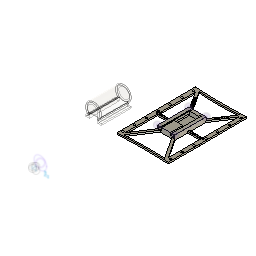
Removeable+Cap (Autodesk Fusion 360 design; units mm, degrees)
Autodesk Fusion 360 part; units mm, degrees
sketch "Sketch1" plane through (0, 0, 0) normal (0, 0, 1) x (1, 0, 0) in component "Base"
  line L0 (65.3388, 0.0001) -> (64.555, 99.997)
  arc A0 (65.3388, 0.0001) -> (0, 0) centre (32.67, -527.6145) ccw
  arc A1 (58.214, 2.2762) -> (6.5482, 1.9998) centre (35.1249, -510.6694) ccw
  arc A2 (-0.7816, 100.3921) -> (64.555, 99.997) centre (35.0771, 627.7997) ccw
  arc A3 (6.5746, 97.8855) -> (58.214, 97.7209) centre (33.5966, 474.9447) ccw
  line L1 (-0.4188, 49.9985) -> (5, 50.0245) construction
  circle A4 centre (2.2906, 50.0115) radius 1.25
  line L2 (4.7824, 95.0143) -> (-0.2636, 95.0087) construction
  circle A5 centre (2.2594, 95.0115) radius 1.25
  line L3 (2.2906, 50.0115) -> (2.274, 65.0115) construction
  line L4 (2.274, 65.0115) -> (2.2574, 80.0115) construction
  line L5 (2.2574, 80.0115) -> (2.2594, 95.0115) construction
  circle A6 centre (2.2574, 80.0115) radius 1.25
  circle A7 centre (2.274, 65.0115) radius 1.25
  circle A8 centre (62.7399, 95.0115) radius 1.25
  circle A9 centre (62.7419, 80.0115) radius 1.25
  circle A10 centre (62.7253, 65.0115) radius 1.25
  circle A11 centre (62.7087, 50.0115) radius 1.25
  circle A12 centre (62.7253, 35.0115) radius 1.25
  circle A13 centre (62.7419, 20.0115) radius 1.25
  circle A14 centre (62.7399, 5.0116) radius 1.25
  circle A15 centre (2.2594, 5.0116) radius 1.25
  circle A16 centre (2.2574, 20.0115) radius 1.25
  circle A17 centre (2.274, 35.0115) radius 1.25
  line L6 (-0.7816, 100.3921) -> (0, 0)
  line L7 (60.0224, 46.1) -> (60.0224, 5.0699)
  line L8 (5, 5) -> (5, 46.2745)
  line L9 (2.2574, 80.0115) -> (2.2576, 81.0115)
  line L10 (60.0224, 97.8257) -> (60.0224, 2.1916)
  line L11 (60.0224, 46.1) -> (60.0224, 48.6)
  line L12 (65.0224, 100) -> (65.0224, 0)
  line L13 (40.775, 30.0973) -> (72.9042, 30.0973) construction
  line L14 (60.0224, 2.1916) -> (61.5224, 2.1916) construction
  line L15 (60.0224, 2.1916) -> (61.5224, 2.1916) construction
  line L16 (58.214, 2.2762) -> (39.7178, 30.0973)
  line L17 (4.9833, 2.4465) -> (5, 2.4465) construction
  line L18 (24.6632, 30.0973) -> (6.5482, 1.9998)
  line L19 (58.214, 97.7209) -> (39.8492, 70.0973)
  line L20 (60.0224, 94.9271) -> (43.275, 69.7364)
  line L21 (24.6894, 70.0973) -> (6.5, 98)
  line L22 (5, 94.8639) -> (21.275, 69.5842)
  line L23 (64.9469, 49.9985) -> (-0.4188, 49.9985) construction
  line L24 (5, 50.0245) -> (5.0001, 49.9985)
  line L25 (5.0001, 49.9985) -> (5, 50.0245)
  line L26 (5.006, 48.7745) -> (21.275, 48.7745)
  line L27 (5, 51.2745) -> (4.994, 51.2745)
  line L28 (60.0224, 50.0087) -> (60.0224, 49.9985)
  line L29 (60.0224, 48.7587) -> (43.275, 48.9043)
  line L30 (60.0224, 94.9271) -> (60.0224, 51.2587)
  line L31 (60.0224, 48.7587) -> (60.0224, 48.6)
  line L32 (5, 49.9985) -> (5, 50.0245)
  line L33 (5, 51.2745) -> (5, 94.8639)
  line L34 (43.275, 46.4131) -> (60.0229, 46.4131)
  line L35 (60.0224, 51.2587) -> (60.0224, 48.7587)
  line L36 (21.275, 46.2745) -> (5, 46.2745)
  line L37 (4.994, 51.2745) -> (5.006, 48.7745)
  line L38 (39.8492, 70.0973) -> (24.6894, 70.0973)
  line L39 (24.6632, 30.0973) -> (39.7178, 30.0973)
  line L40 (43.275, 70.0973) -> (32.2207, 49.9985) construction
  line L41 (5, 5) -> (21.275, 30.2436)
  line L42 (60.0224, 5.0699) -> (43.275, 30.2607)
  line L43 (21.275, 70.0973) -> (32.3293, 49.9985) construction
  line L44 (21.275, 69.5842) -> (21.275, 48.7745)
  line L45 (21.275, 46.2745) -> (21.275, 30.2436)
  line L46 (43.275, 30.2607) -> (43.275, 46.4131)
  line L47 (43.275, 48.9043) -> (43.275, 69.7364)
  line L48 (43.275, 30.0973) -> (21.275, 30.0973)
  line L49 (21.275, 30.0973) -> (21.275, 70.0973)
  line L50 (21.275, 70.0973) -> (43.275, 70.0973)
  line L51 (43.275, 70.0973) -> (43.275, 30.0973)
  line L52 (43.275, 30.0973) -> (21.275, 70.0973) construction
  line L53 (21.275, 30.0973) -> (43.275, 70.0973) construction
  point P0 (32.275, 50.0973)
  point P1 (32.275, 50.0973)
  point P2 (32.275, 50.0973)
  point P3 (32.275, 50.0973)
  point P4 (32.275, 50.0973)
  dimension "d2" = 2.5
  dimension "d4" = 2.5
  dimension "d7" = 2.5
  dimension "d8" = 2.5
  dimension "d13" = 100
  dimension "d192" = 2.5
  dimension "d209" = 1
  dimension "d218" = 5
  dimension "d384" = 22
  dimension "d385" = 40
  constraint vertical L8
  constraint vertical L30
  constraint coincident A0.end L6.end
  constraint coincident L1.end L8
  constraint midpoint L1 A4.centre
  constraint midpoint L2 A5.centre
  constraint coincident A4.centre L3.start
  constraint perpendicular L2 L3
  constraint perpendicular L2 L4
  constraint coincident A5.centre L5.end
  constraint coincident L4.end L5.start
  constraint coincident L3.end L4.start
  constraint collinear L7 L30
  constraint collinear L8 L32
  constraint parallel L5 L9
  constraint coincident L10.end L14.start
  constraint horizontal L13
  constraint horizontal L14
  constraint horizontal L15
  constraint parallel L16 L42
  constraint horizontal L17
  constraint parallel L18 L41
  constraint coincident L21 A3.start
  constraint coincident P4 P3
  constraint midpoint L0 L23.start
  constraint horizontal L23
  constraint perpendicular L1 L24
  constraint perpendicular L1 L25
  constraint midpoint L10 L28.start
  constraint parallel L11 L28
  constraint collinear L30 L31
  constraint coincident L23 L28.end
  constraint coincident L23 L32.start
  constraint collinear L32 L33
  constraint coincident L23 L24.end
  constraint horizontal L34
  constraint horizontal L38
  constraint perpendicular L38 L44
  constraint parallel L38 L39
  constraint parallel L44 L46
  constraint coincident L40 P4
  constraint coincident P4 L43
  constraint coincident L23 L40.end
  constraint coincident L23 L43.end
  constraint coincident L36.start L44
  constraint coincident L29.end L46
  constraint collinear L44 L45
  constraint collinear L46 L47
  constraint horizontal L48
  constraint perpendicular L48 L49
  constraint parallel L48 L50
  constraint parallel L49 L51
  constraint coincident L52 P4
  constraint coincident L53 P4
  measures "d2" diameter of A4
  measures "d4" diameter of A5
  measures "d7" diameter of A6
  measures "d8" diameter of A7
  measures "d13" distance of L0.start L0.end
  measures "d192" diameter of A5
  measures "d209" distance of L4.end L9.end
  measures "d218" distance of L7 L12
  measures "d384" distance of L43.start L40.start
  measures "d385" distance of L48.end L43.start
extrude "Extrude1" add sketch "Sketch1" along normal blind 6 contours L38 L39 L44 L45 L46 L47 L48 L49 L50 L51 makes body 1 in component "Base"
extrude "Extrude2" add sketch "Sketch1" along normal blind 2 separate body contours L0 A0 A2 L6 L12 | L38 L39 L44 L45 L46 L47 L48 L49 L50 L51 | L10 L11 L29 L31 L34 L51 makes body 2 in component "Base"
sketch "Sketch9" plane through (0, 0, 6) normal (0, 0, 1) x (-1, 0, 0) in component "Base"
  line L0 (-23.462, -48.6115) -> (-22.275, -48.6115)
  line L1 (-32.4463, -66.0115) -> (-27.1964, -65.9812)
  line L2 (-27.1964, -65.9812) -> (-37.6964, -65.9812)
  line L3 (-23.462, -48.6115) -> (-25.9464, -48.6115)
  line L4 (-26.9547, -45.9812) -> (-22.275, -45.9812)
  line L5 (-42.275, -48.6115) -> (-38.9464, -48.6115)
  line L6 (-37.9464, -45.9812) -> (-42.275, -45.9812)
  line L7 (-42.2726, -46.1115) -> (-42.2726, -48.6115)
  line L8 (-22.275, -30.0973) -> (-42.275, -30.0973)
  line L9 (-42.275, -70.0973) -> (-22.275, -70.0973)
  line L10 (-22.462, -48.6115) -> (-22.4997, -48.6115)
  line L11 (-42.275, -48.6115) -> (-42.275, -45.9812)
  line L12 (-37.9464, -45.9812) -> (-26.9547, -45.9812)
  line L13 (-26.9464, -65.9812) -> (-37.9464, -65.9812)
  line L14 (-42.275, -70.0973) -> (-42.275, -69.0973)
  line L15 (-43.275, -70.0973) -> (-21.275, -70.0973)
  line L16 (-21.275, -70.0973) -> (-21.275, -30.0973)
  line L17 (-21.275, -30.0973) -> (-43.275, -30.0973)
  line L18 (-43.275, -30.0973) -> (-43.275, -70.0973)
  line L19 (-43.275, -70.0973) -> (-21.275, -70.0973)
  line L20 (-21.275, -70.0973) -> (-21.275, -30.0973)
  line L21 (-21.275, -30.0973) -> (-43.275, -30.0973)
  line L22 (-43.275, -30.0973) -> (-43.275, -70.0973)
  line L23 (-22.275, -45.9812) -> (-22.275, -48.6115)
  line L24 (-26.9464, -65.9812) -> (-25.9464, -65.9812)
  line L25 (-37.9464, -65.9812) -> (-38.9464, -65.9812)
  line L26 (-38.9464, -65.9812) -> (-38.9464, -45.9812)
  line L27 (-25.9464, -65.9812) -> (-25.9464, -45.9812)
  dimension "d179" = 11
  dimension "d308" = 20
  dimension "d337" = 1
  dimension "d386" = 1
  dimension "d390" = 1
  dimension "d391" = 1
  dimension "d392" = 1
  dimension "d393" = 1
  constraint horizontal L2
  constraint horizontal L3
  constraint horizontal L4
  constraint horizontal L5
  constraint horizontal L6
  constraint vertical L7
  constraint perpendicular L6 L11
  constraint coincident L9.start L14.start
  constraint coincident L6 L26.end
  constraint perpendicular L6 L26
  constraint perpendicular L24 L27
  constraint coincident L26 L5.end
  constraint coincident L27 L3.end
  constraint coincident L4 L27.end
  constraint perpendicular L4 L27
  measures "d179" distance of L13.start L13.end
  measures "d308" distance of L2 L12
  measures "d337" distance of L9.start L14.end
  measures "d386" distance of L11 L18
  measures "d390" distance of L0.end L16
  measures "d391" distance of L4.end L16
  measures "d392" distance of L13.start L24.end
  measures "d393" distance of L13.end L25.end
sketch "Sketch5" plane through (0, 0, 6) normal (0, 0, 1) x (-1, 0, 0)
  line L0 (-43.275, -70.0973) -> (-21.275, -70.0973)
  line L1 (-21.275, -70.0973) -> (-21.275, -30.0973)
  line L2 (-21.275, -30.0973) -> (-43.275, -30.0973)
  line L3 (-43.275, -30.0973) -> (-43.275, -70.0973)
move_body "Move1" bodies 2 1 to x (1, 0, 0) y (0, 1, 0) z (0, 0, 1) at (-32.275, -50.0973, 0) in component "Base"
combine "Combine5" operation add target body 2 tool bodies 1 in component "Base"
move_body "Move2" bodies 2 to x (1, 0, 0) y (0, 1, 0) z (0, 0, 1) at (32.275, 50.0973, 0) in component "Base"
extrude "Extrude3" cut sketch "Sketch9" against normal blind 5 contours L2 L4 L6 L12 L13 L24 L25 L26 L27 bodies 2 in component "Base"
extrude "Extrude5" cut sketch "Sketch9" against normal blind 4.5 from surface at -1 contours L0 L3 L4 L10 L23 L27 | L5 L6 L11 L26 bodies 2 in component "Base"
sketch "Sketch13" plane through (0, 0, 2) normal (0, 0, 1) x (-1, 0, 0) in component "Base"
  circle A0 centre (-2.2594, -95.0115) radius 1.25
  circle A1 centre (-2.274, -65.0115) radius 1.25
  circle A2 centre (-2.2574, -80.0115) radius 1.25
  circle A3 centre (-2.2574, -20.0115) radius 1.25
  circle A4 centre (-2.274, -35.0115) radius 1.25
  circle A5 centre (-62.7419, -20.0115) radius 1.25
  circle A6 centre (-62.7087, -50.0115) radius 1.25
  circle A7 centre (-62.7419, -80.0115) radius 1.25
  circle A8 centre (-62.7253, -35.0115) radius 1.25
  circle A9 centre (-62.7399, -95.0115) radius 1.25
  circle A10 centre (-62.7253, -65.0115) radius 1.25
  circle A11 centre (-62.7399, -5.0116) radius 1.25
  line L0 (-6.5482, -1.9998) -> (-24.6632, -30.0973)
  line L1 (-24.6632, -30.0973) -> (-22.275, -30.0973)
  line L2 (-4.994, -51.2745) -> (-5, -51.2745)
  line L3 (-5, -51.2745) -> (-5, -94.8639)
  line L4 (-5, -94.8639) -> (-22.275, -68.0309)
  line L5 (-22.275, -68.0309) -> (-22.275, -70.0973)
  line L6 (-22.275, -70.0973) -> (-24.6894, -70.0973)
  line L7 (-24.6894, -70.0973) -> (-6.5746, -97.8855)
  line L8 (-58.214, -97.7209) -> (-39.8492, -70.0973)
  line L9 (-39.8492, -70.0973) -> (-42.275, -70.0973)
  line L10 (-42.275, -70.0973) -> (-42.275, -68.2322)
  line L11 (-42.275, -68.2322) -> (-60.0224, -94.9271)
  line L12 (-60.0224, -94.9271) -> (-60.0224, -48.7587)
  line L13 (-60.0224, -48.7587) -> (-42.275, -48.913)
  line L14 (-42.275, -48.913) -> (-42.275, -46.4131)
  line L15 (-42.275, -46.4131) -> (-60.0224, -46.4131)
  line L16 (-60.0224, -46.4131) -> (-60.0224, -5.0699)
  line L17 (-42.275, -30.0973) -> (-39.7178, -30.0973)
  line L18 (-39.7178, -30.0973) -> (-58.214, -2.2762)
  circle A12 centre (-2.2594, -5.0116) radius 1.25
  circle A13 centre (-2.2906, -50.0115) radius 1.25
  line L19 (-65.0224, -40.3697) -> (-64.555, -99.997)
  line L20 (0.7816, -100.3921) -> (0, 0)
  circle A14 centre (-2.2594, -95.0115) radius 1.25
  circle A15 centre (-2.274, -65.0115) radius 1.25
  circle A16 centre (-2.2574, -80.0115) radius 1.25
  circle A17 centre (-2.2574, -20.0115) radius 1.25
  circle A18 centre (-2.274, -35.0115) radius 1.25
  circle A19 centre (-62.7419, -20.0115) radius 1.25
  circle A20 centre (-62.7087, -50.0115) radius 1.25
  circle A21 centre (-62.7419, -80.0115) radius 1.25
  circle A22 centre (-62.7253, -35.0115) radius 1.25
  circle A23 centre (-62.7399, -95.0115) radius 1.25
  circle A24 centre (-62.7253, -65.0115) radius 1.25
  circle A25 centre (-62.7399, -5.0116) radius 1.25
  line L21 (-6.5482, -1.9998) -> (-24.6632, -30.0973)
  line L22 (-4.994, -51.2745) -> (-5, -51.2745)
  line L23 (-5, -51.2745) -> (-5, -94.8639)
  line L24 (-5, -94.8639) -> (-21.275, -69.5842)
  line L25 (-24.6894, -70.0973) -> (-6.5746, -97.8855)
  line L26 (-58.214, -97.7209) -> (-39.8492, -70.0973)
  line L27 (-43.275, -69.7364) -> (-60.0224, -94.9271)
  line L28 (-60.0224, -94.9271) -> (-60.0224, -48.7587)
  line L29 (-60.0224, -48.7587) -> (-43.275, -48.9043)
  line L30 (-43.275, -46.4131) -> (-60.0224, -46.4131)
  line L31 (-60.0224, -46.4131) -> (-60.0224, -5.0699)
  line L32 (-39.7178, -30.0973) -> (-58.214, -2.2762)
  arc A26 (-58.214, -2.2762) -> (-6.5482, -1.9998) centre (-35.1249, 510.6694) ccw
  circle A27 centre (-2.2594, -5.0116) radius 1.25
  circle A28 centre (-2.2906, -50.0115) radius 1.25
  line L33 (-65.0224, -40.3697) -> (-64.555, -99.997)
  line L34 (0.7816, -100.3921) -> (0, 0)
  arc A29 (-65.0224, -0.0196) -> (0, 0) centre (-32.67, 527.6145) ccw
  line L35 (-65.0224, -0.0196) -> (-65.0224, -40.3697)
  line L36 (-60.0224, -47.5859) -> (-38, -47.5859)
  line L37 (-5.003, -47.5245) -> (-26.9697, -47.4718)
  line L38 (-5.003, -47.5245) -> (-3.003, -47.5293)
  line L39 (-60.0224, -47.5859) -> (-62.0223, -47.6016)
  line L40 (-24.6632, -30.0973) -> (-21.275, -30.0973)
  line L41 (-21.275, -30.0973) -> (-21.275, -30.2436)
  line L42 (-21.275, -46.2745) -> (-21.275, -48.7745)
  line L43 (-21.275, -69.5842) -> (-21.275, -70.0973)
  line L44 (-21.275, -70.0973) -> (-24.6894, -70.0973)
  line L45 (-39.8492, -70.0973) -> (-43.275, -70.0973)
  line L46 (-43.275, -70.0973) -> (-43.275, -69.7364)
  line L47 (-43.275, -48.9043) -> (-43.275, -46.4131)
  line L48 (-43.275, -30.2607) -> (-43.275, -30.0973)
  line L49 (-43.275, -30.0973) -> (-39.7178, -30.0973)
  dimension "d252" = 2
  dimension "d253" = 2
  constraint parallel L37 L38
  constraint perpendicular L19 L39
  measures "d252" distance of L37.start L38.end
  measures "d253" distance of L36.start L39.end
pipe "Pipe9" cut diameter 1.5 path "Sketch13" along L39 L36 bodies 2 in component "Base"
pipe "Pipe10" cut diameter 1.5 path "Sketch13" along L37 L38 bodies 2 in component "Base"
sketch "Sketch3" plane through (0, 0, 2) normal (0, 0, 1) x (-1, 0, 0)
  circle A0 centre (-2.2594, -95.0115) radius 1.25
  circle A1 centre (-2.274, -65.0115) radius 1.25
  circle A2 centre (-2.2574, -80.0115) radius 1.25
  circle A3 centre (-2.2574, -20.0115) radius 1.25
  circle A4 centre (-2.274, -35.0115) radius 1.25
  circle A5 centre (-62.7419, -20.0115) radius 1.25
  circle A6 centre (-62.7087, -50.0115) radius 1.25
  circle A7 centre (-62.7419, -80.0115) radius 1.25
  circle A8 centre (-62.7253, -35.0115) radius 1.25
  circle A9 centre (-62.7399, -95.0115) radius 1.25
  circle A10 centre (-62.7253, -65.0115) radius 1.25
  circle A11 centre (-62.7399, -5.0116) radius 1.25
  line L0 (-21.275, -46.7355) -> (-3.0012, -46.7793)
  line L1 (-3.0012, -46.7793) -> (-3.0048, -48.2793)
  line L2 (-3.0048, -48.2793) -> (-21.275, -48.2355)
  line L3 (-21.275, -48.7745) -> (-5.006, -48.7745)
  line L4 (-5.006, -48.7745) -> (-4.994, -51.2745)
  line L5 (-4.994, -51.2745) -> (-5, -51.2745)
  line L6 (-5, -51.2745) -> (-5, -94.8639)
  line L7 (-5, -94.8639) -> (-21.275, -69.5842)
  line L8 (-24.6894, -70.0973) -> (-6.5746, -97.8855)
  arc A12 (-6.5746, -97.8855) -> (-58.214, -97.7209) centre (-33.5966, -474.9447) ccw
  line L9 (-58.214, -97.7209) -> (-39.8492, -70.0973)
  line L10 (-43.275, -69.7364) -> (-60.0224, -94.9271)
  line L11 (-60.0224, -94.9271) -> (-60.0224, -48.7587)
  line L12 (-60.0224, -48.7587) -> (-43.275, -48.9043)
  line L13 (-43.275, -48.3359) -> (-60.0165, -48.3359)
  line L14 (-60.0165, -48.3359) -> (-62.0165, -48.3516)
  line L15 (-62.0165, -48.3516) -> (-62.0282, -46.8516)
  line L16 (-62.0282, -46.8516) -> (-60.0283, -46.8359)
  line L17 (-60.0222, -46.8359) -> (-43.275, -46.8359)
  line L18 (-43.275, -46.4131) -> (-60.0224, -46.4131)
  line L19 (-60.0224, -46.4131) -> (-60.0224, -5.0699)
  line L20 (-60.0224, -5.0699) -> (-43.275, -30.2607)
  line L21 (-39.7178, -30.0973) -> (-58.214, -2.2762)
  arc A13 (-58.214, -2.2762) -> (-6.5482, -1.9998) centre (-35.1249, 510.6694) ccw
  line L22 (-6.5482, -1.9998) -> (-24.6632, -30.0973)
  line L23 (-21.275, -30.2436) -> (-5, -5)
  line L24 (-5, -5) -> (-5, -46.2745)
  line L25 (-5, -46.2745) -> (-21.275, -46.2745)
  circle A14 centre (-2.2594, -5.0116) radius 1.25
  circle A15 centre (-2.2906, -50.0115) radius 1.25
  line L26 (-65.0224, -40.3697) -> (-64.555, -99.997)
  arc A16 (0.7816, -100.3921) -> (-64.555, -99.997) centre (-35.0771, -627.7997) ccw
  line L27 (0.7816, -100.3921) -> (0, 0)
  arc A17 (-65.0224, -0.0196) -> (0, 0) centre (-32.67, 527.6145) ccw
  line L28 (-65.0224, -0.0196) -> (-65.0224, -40.3697)
  line L29 (-51.9391, -88.7994) -> (-42.8906, -75.8768) construction
  line L30 (-42.8906, -75.8768) -> (-45.367, -74.1428) construction
  line L31 (-45.367, -74.1428) -> (-54.4155, -87.0654) construction
  line L32 (-54.4155, -87.0654) -> (-51.9391, -88.7994) construction
  line L33 (-23.0791, -75.4122) -> (-12.4993, -91.7036) construction
  line L34 (-12.4993, -91.7036) -> (-8.9525, -89.4003) construction
  line L35 (-8.9525, -89.4003) -> (-19.5323, -73.1089) construction
  line L36 (-19.5323, -73.1089) -> (-23.0791, -75.4122) construction
  line L37 (-21.275, -48.2355) -> (-21.275, -48.7745)
  line L38 (-21.275, -69.5842) -> (-21.275, -70.0973)
  line L39 (-21.275, -70.0973) -> (-24.6894, -70.0973)
  line L40 (-39.8492, -70.0973) -> (-43.275, -70.0973)
  line L41 (-43.275, -70.0973) -> (-43.275, -69.7364)
  line L42 (-43.275, -48.9043) -> (-43.275, -48.3359)
  line L43 (-43.275, -46.8359) -> (-43.275, -46.4131)
  line L44 (-43.275, -30.2607) -> (-43.275, -30.0973)
  line L45 (-43.275, -30.0973) -> (-39.7178, -30.0973)
  line L46 (-24.6632, -30.0973) -> (-21.275, -30.0973)
  line L47 (-21.275, -30.0973) -> (-21.275, -30.2436)
  line L48 (-21.275, -46.2745) -> (-21.275, -46.7355)
  dimension "d256" = 2
  dimension "d258" = 2
sketch "Sketch14" plane through (0, 0, 2) normal (0, 0, 1) x (-1, 0, 0) in component "Base"
  circle A0 centre (-2.2594, -95.0115) radius 1.25
  circle A1 centre (-2.274, -65.0115) radius 1.25
  circle A2 centre (-2.2574, -80.0115) radius 1.25
  circle A3 centre (-2.2574, -20.0115) radius 1.25
  circle A4 centre (-2.274, -35.0115) radius 1.25
  circle A5 centre (-62.7419, -20.0115) radius 1.25
  circle A6 centre (-62.7087, -50.0115) radius 1.25
  circle A7 centre (-62.7419, -80.0115) radius 1.25
  circle A8 centre (-62.7253, -35.0115) radius 1.25
  circle A9 centre (-62.7399, -95.0115) radius 1.25
  circle A10 centre (-62.7253, -65.0115) radius 1.25
  circle A11 centre (-62.7399, -5.0116) radius 1.25
  line L0 (-21.275, -46.7355) -> (-3.0012, -46.7793)
  line L1 (-3.0012, -46.7793) -> (-3.0048, -48.2793)
  line L2 (-3.0048, -48.2793) -> (-21.275, -48.2355)
  line L3 (-21.275, -48.7745) -> (-5.006, -48.7745)
  line L4 (-5.006, -48.7745) -> (-4.994, -51.2745)
  line L5 (-4.994, -51.2745) -> (-5, -51.2745)
  line L6 (-5, -51.2745) -> (-5, -94.8639)
  line L7 (-5, -94.8639) -> (-21.275, -69.5842)
  line L8 (-24.6894, -70.0973) -> (-6.5746, -97.8855)
  arc A12 (-6.5746, -97.8855) -> (-58.214, -97.7209) centre (-33.5966, -474.9447) ccw
  line L9 (-58.214, -97.7209) -> (-39.8492, -70.0973)
  line L10 (-43.275, -69.7364) -> (-60.0224, -94.9271)
  line L11 (-60.0224, -94.9271) -> (-60.0224, -48.7587)
  line L12 (-60.0224, -48.7587) -> (-43.275, -48.9043)
  line L13 (-43.275, -48.3359) -> (-60.0165, -48.3359)
  line L14 (-60.0165, -48.3359) -> (-62.0165, -48.3516)
  line L15 (-62.0165, -48.3516) -> (-62.0282, -46.8516)
  line L16 (-62.0282, -46.8516) -> (-60.0283, -46.8359)
  line L17 (-60.0222, -46.8359) -> (-43.275, -46.8359)
  line L18 (-43.275, -46.4131) -> (-60.0224, -46.4131)
  line L19 (-60.0224, -46.4131) -> (-60.0224, -5.0699)
  line L20 (-60.0224, -5.0699) -> (-43.275, -30.2607)
  line L21 (-39.7178, -30.0973) -> (-58.214, -2.2762)
  arc A13 (-58.214, -2.2762) -> (-6.5482, -1.9998) centre (-35.1249, 510.6694) ccw
  line L22 (-6.5482, -1.9998) -> (-24.6632, -30.0973)
  line L23 (-21.275, -30.2436) -> (-5, -5)
  line L24 (-5, -5) -> (-5, -46.2745)
  line L25 (-5, -46.2745) -> (-21.275, -46.2745)
  circle A14 centre (-2.2594, -5.0116) radius 1.25
  circle A15 centre (-2.2906, -50.0115) radius 1.25
  line L26 (-65.0224, -40.3697) -> (-64.555, -99.997)
  arc A16 (0.7816, -100.3921) -> (-64.555, -99.997) centre (-35.0771, -627.7997) ccw
  line L27 (0.7816, -100.3921) -> (0, 0)
  arc A17 (-65.0224, -0.0196) -> (0, 0) centre (-32.67, 527.6145) ccw
  line L28 (-65.0224, -0.0196) -> (-65.0224, -40.3697)
  line L29 (-51.9391, -88.7994) -> (-42.8906, -75.8768) construction
  line L30 (-42.8906, -75.8768) -> (-45.367, -74.1428) construction
  line L31 (-45.367, -74.1428) -> (-54.4155, -87.0654) construction
  line L32 (-54.4155, -87.0654) -> (-51.9391, -88.7994) construction
  line L33 (-23.0791, -75.4122) -> (-12.4993, -91.7036) construction
  line L34 (-12.4993, -91.7036) -> (-8.9525, -89.4003) construction
  line L35 (-8.9525, -89.4003) -> (-19.5323, -73.1089) construction
  line L36 (-19.5323, -73.1089) -> (-23.0791, -75.4122) construction
  line L37 (-21.275, -48.2355) -> (-21.275, -48.7745)
  line L38 (-21.275, -69.5842) -> (-21.275, -70.0973)
  line L39 (-21.275, -70.0973) -> (-24.6894, -70.0973)
  line L40 (-39.8492, -70.0973) -> (-43.275, -70.0973)
  line L41 (-43.275, -70.0973) -> (-43.275, -69.7364)
  line L42 (-43.275, -48.9043) -> (-43.275, -48.3359)
  line L43 (-43.275, -46.8359) -> (-43.275, -46.4131)
  line L44 (-43.275, -30.2607) -> (-43.275, -30.0973)
  line L45 (-43.275, -30.0973) -> (-39.7178, -30.0973)
  line L46 (-24.6632, -30.0973) -> (-21.275, -30.0973)
  line L47 (-21.275, -30.0973) -> (-21.275, -30.2436)
  line L48 (-21.275, -46.2745) -> (-21.275, -46.7355)
  dimension "d259" = 2
  dimension "d260" = 2
  text T0 "BILBY" font "Arial" height 2 align left top in box 15.7756 x 3.023 at (-51.9391, -88.7994) x (0.573576, 0.819152) y (-0.819152, 0.573576) spacing 2 kerned
  text T1 "ROCKET\n" font "Arial" height 2 align left top in box 19.4253 x 4.229 at (-23.0791, -75.4122) x (0.544639, -0.838671) y (0.838671, 0.544639) spacing 2 kerned
emboss "Emboss3" depth 0.5 profiles "Sketch14" section 1 text T0 onto face at (62.3819, 40.959, 2) on bodies 2 bodies 2 in component "Base"
emboss "Emboss4" depth 0.5 profiles "Sketch14" section 1 text T1 onto face at (62.3819, 40.959, 2) on bodies 2 bodies 2 in component "Base"
sketch "Sketch1 (2)" plane through (0, 0, 0) normal (1, 0, 0) x (0, 1, 0) in component "Removable Lid"
  line L0 (-78.5866, 26.583) -> (-60.5866, 26.583)
  line L1 (-59.5941, 25.583) -> (-59.5866, 25.583)
  line L2 (-58.5851, 24.3344) -> (-58.5851, 17.5829)
  arc A0 (-59.5866, 25.583) -> (-60.5866, 26.583) centre (-60.5866, 25.583) ccw
  arc A1 (-58.5862, 26.5834) -> (-59.5862, 27.583) centre (-59.5862, 26.583) ccw
  line L3 (-59.5866, 25.583) -> (-59.5866, 17.5829)
  line L4 (-98.5867, 27.583) -> (-98.5866, 27.583)
  line L5 (-58.585, 24.0834) -> (-58.5851, 24.3344)
  line L6 (-58.585, 24.0834) -> (-58.5862, 26.5834)
  line L7 (-78.5866, 27.583) -> (-59.5862, 27.583)
  line L8 (-97.5866, 25.583) -> (-97.5866, 17.5829)
  line L9 (-98.5881, 24.3344) -> (-98.5881, 17.5829)
  line L10 (-97.5792, 25.583) -> (-97.5866, 25.583)
  arc A2 (-96.5866, 26.583) -> (-97.5866, 25.583) centre (-96.5866, 25.583) ccw
  line L11 (-98.5882, 24.0834) -> (-98.5881, 24.3344)
  line L12 (-78.5866, 27.583) -> (-97.5871, 27.583)
  arc A3 (-97.5871, 27.583) -> (-98.5871, 26.5834) centre (-97.5871, 26.583) ccw
  line L13 (-78.5866, 26.583) -> (-96.5866, 26.583)
  line L14 (-98.5882, 24.0834) -> (-98.5871, 26.5834)
  line L15 (-98.5881, 17.5829) -> (-97.5866, 17.5829)
  line L16 (-59.5866, 17.5829) -> (-58.5851, 17.5829)
  line L17 (-59.5866, 17.5829) -> (-97.5866, 17.5829) construction
  line L18 (-59.5941, 25.583) -> (-58.5862, 26.5834)
  line L19 (-97.5792, 25.583) -> (-98.5871, 26.5834)
  point P0 (-59.5866, 26.583)
  point P1 (-58.5866, 27.583)
  point P2 (-78.5866, 17.583)
  point P3 (-78.5866, 17.583)
  point P4 (-98.5866, 27.583)
  point P5 (-97.5866, 26.583)
  dimension "d309" = 40
  dimension "d311" = 10
  dimension "d312" = 19
  dimension "d316" = 1
  dimension "d317" = 1
  constraint coincident P3 P2
  constraint vertical L3
  constraint parallel L5 L6
  constraint coincident P1 L6
  constraint tangent A1 L6
  constraint coincident P0 L0
  constraint coincident P0 L3
  constraint tangent L0 A0
  constraint tangent A0 L3
  constraint tangent A1 L7
  constraint perpendicular L2 L16
  constraint perpendicular L8 L17
  measures "d309" distance of P4 P1
  measures "d311" distance of P3 L7.start
  measures "d312" distance of L0.start P0
  measures "d316" radius of A1
  measures "d317" radius of A0
revolve "Revolve1" add sketch "Sketch1 (2)" angle 143 about axis through (0, -59.5866, 17.5829) along (0, 1, 0) second angle 143 separate body contours L0 A0 A1 L7 A2 L12 A3 L13 L18 L19 makes body 3 in component "Removable Lid"
revolve "Revolve2" add sketch "Sketch1 (2)" angle 360 about axis through (0, -59.5866, 17.5829) along (0, -1, 0) contours L8 L9 A2 L11 L14 L15 L19 bodies 3 in component "Removable Lid"
revolve "Revolve3" add sketch "Sketch1 (2)" angle 360 about axis through (0, -59.5866, 17.5829) along (0, -1, 0) contours L2 A0 L3 L5 L6 L16 L18 bodies 3 in component "Removable Lid"
sketch "Sketch7" plane through (0, -97.5866, 0) normal (0, 1, 0) x (-1, 0, 0) in component "Removable Lid"
  circle A0 centre (0, 17.5829) radius 8
  line L0 (-5.5, 3.5) -> (5.5, 3.5)
  line L1 (5.5, 3.5) -> (5.5, 13.5)
  line L2 (5.5, 13.5) -> (-5.5, 13.5)
  line L3 (-5.5, 13.5) -> (-5.5, 3.5)
  line L4 (-5.5, 3.5) -> (5.5, 13.5) construction
  line L5 (5.5, 3.5) -> (-5.5, 13.5) construction
  line L6 (-5.25, 3.9) -> (5.25, 3.9)
  line L7 (5.25, 3.9) -> (5.25, 13.1)
  line L8 (5.25, 13.1) -> (-5.25, 13.1)
  line L9 (-5.25, 13.1) -> (-5.25, 3.9)
  line L10 (-5.25, 3.9) -> (5.25, 13.1) construction
  line L11 (5.25, 3.9) -> (-5.25, 13.1) construction
  point P0 (0, 8.5)
  point P1 (0, 8.5)
  dimension "d396" = 11
  dimension "d397" = 10
  dimension "d398" = 10.5
  dimension "d399" = 9.2
  constraint horizontal L0
  constraint perpendicular L0 L1
  constraint parallel L0 L2
  constraint parallel L1 L3
  constraint coincident L4 P1
  constraint coincident L5 P1
  constraint horizontal L6
  constraint perpendicular L6 L7
  constraint parallel L6 L8
  constraint parallel L7 L9
  constraint coincident L10 P1
  constraint coincident L11 P1
  constraint coincident P1 P0
  measures "d396" distance of L1.end L2.end
  measures "d397" distance of L0.end L1.end
  measures "d398" distance of L7.end L8.end
  measures "d399" distance of L6.end L7.end
sketch "Sketch4" plane through (0, -97.5866, 0) normal (0, -1, 0) x (1, 0, 0) in component "Removable Lid"
  line L0 (-7, 10.3227) -> (-6.468, 11.113)
  line L1 (-6.468, 11.113) -> (-5.5, 11.113)
  line L2 (-7, 10.3227) -> (-7, 8.3227)
  line L3 (-7, 8.3227) -> (-10, 8.3227)
  line L4 (-10, 8.3227) -> (-10, 6.3227)
  line L5 (-10, 6.3227) -> (-5.5, 6.3227)
  line L6 (-5.5, 6.3227) -> (-5.5, 11.113)
  circle A0 centre (0, 17.5829) radius 8
  line L7 (7, 10.213) -> (6.5, 11.113)
  line L8 (7, 10.213) -> (7, 8.213)
  line L9 (7, 8.213) -> (10, 8.213)
  line L10 (10, 8.213) -> (10, 6.213)
  line L11 (10, 6.213) -> (5.5, 6.213)
  line L12 (5.5, 6.213) -> (5.5, 11.113)
  line L13 (5.5, 11.113) -> (6.5, 11.113)
  dimension "d367" = 0.9527
  dimension "d368" = 0.968
  dimension "d369" = 2
  dimension "d370" = 3
  dimension "d371" = 2
  dimension "d372" = 4.5
  constraint horizontal L1
  constraint coincident L0 L2.start
  constraint vertical L2
  constraint coincident L2 L3.start
  constraint perpendicular L2 L3
  constraint coincident L3 L4.start
  constraint perpendicular L3 L4
  constraint coincident L4 L5.start
  constraint perpendicular L4 L5
  constraint coincident L5 L6.start
  constraint coincident L1 L6.end
  constraint vertical L6
  constraint vertical L8
  constraint perpendicular L8 L9
  constraint perpendicular L9 L10
  constraint perpendicular L10 L11
  constraint perpendicular L11 L12
  constraint perpendicular L12 L13
  measures "d367" distance of L0.start L0.end
  measures "d368" distance of L0.end L1.end
  measures "d369" distance of L7.start L8.end
  measures "d370" distance of L8.end L9.end
  measures "d371" distance of L9.end L10.end
  measures "d372" distance of L10.end L11.end
extrude "Extrude3'" add sketch "Sketch4" against normal blind 38 contours L7 L8 L9 L10 L11 L12 L13 bodies 3 in component "Removable Lid"
extrude "Extrude4" add sketch "Sketch4" against normal blind 38 contours L0 L1 L2 L3 L4 L5 L6 bodies 3 in component "Removable Lid"
extrude "Extrude6" cut sketch "Sketch7" along normal mid plane 6 contours A0 L1 L2 L3 L7 L8 L9 | A0 L0 L1 L3 L6 L7 L9 | A0 L7 L8 L9 | A0 L6 L7 L9 bodies 3 in component "Removable Lid"
move_body "Move3" bodies 3 to x (1, 0, 0) y (0, 1, 0) z (0, 0, 1) at (-10, 97.5871, -6.213) in component "Removable Lid"
move_body "Move4" bodies 3 to x (1, 0, 0) y (0, 1, 0) z (0, 0, 1) at (-20, 0, 0) in component "Removable Lid"
copy_body "CopyPasteBodies3" bodies 3 makes body 4 in component "Base"
move_body "Move7" bodies 4 to x (-1, 0, 0) y (0, -1, 0) z (0, 0, 1) at (0, 0, 0) in component "Base"
move_body "Move8" bodies 4 to x (1, 0, 0) y (0, 1, 0) z (0, 0, 1) at (1.275, 68.0973, 6) in component "Base"
move_body "Move9" bodies 4 to x (1, 0, 0) y (0, 1, 0) z (0, 0, 1) at (1, 0, -3) in component "Base"
combine "Combine9" operation cut target body 2 tool bodies 4 in component "Base"
component "Base" placed x (1, 0, 0) y (0, 1, 0) z (0, 0, 1) at (0, 0, 0)
component "Removable Lid" placed x (1, 0, 0) y (0, 1, 0) z (0, 0, 1) at (0, 0, 0)
